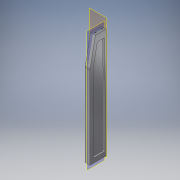
# Autodesk Inventor part: ZcolStiffer
Saved by Autodesk Inventor 2019 (Build 230136000, 136)
## iProperties
Created: 2018-10-03
Part Number: ZcolStiffer
Material: Aluminum 6061-AHC
Document SubType Name: Modeling
Designer: LillaHunden
Density: 2.7 g/cm^3
Appearance: Aluminum - Dark
Mass: 421.378 g
Surface Area: 509.759 cm^2
Volume: 156.066 cm^3
Author: LillaHunden
Autodesk Inventor part; units mm, degrees
ref_plane "YZ Plane" through (0, 0, 0) normal (1, 0, 0) x (0, 1, 0)
ref_plane "XZ Plane" through (0, 0, 0) normal (0, 1, 0) x (-1, 0, 0)
ref_plane "XY Plane" through (0, 0, 0) normal (0, 0, 1) x (1, 0, 0)
ref_plane "Work Plane1" through (0, 0, 0) normal (0, 0, 1) x (1, 0, 0)
sketch "Sketch1" plane through (0, 0, 0) normal (0, 0, 1) x (1, 0, 0)
  line L0 (33.6143, 326.2667) -> (51.0643, 326.2667) construction
  line L1 (0, -13.7333) -> (51.0143, -13.7333) construction
  line L2 (34.8393, 326.2667) -> (49.8393, 326.2667)
  line L3 (49.8393, 326.2667) -> (49.8393, -13.7333)
  line L4 (49.8393, -13.7333) -> (34.8393, -13.7333)
  line L5 (34.8393, -13.7333) -> (34.8393, 326.2667)
  point P0 (0, 0)
  point P1 (51.0143, -13.7333)
  point P2 (42.3393, 326.2667)
  point P3 (42.3393, 326.2667)
  dimension "d0" = 15
  constraints: 8 end point, 2 midpoint, 2 parallel, 1 coincident, 1 horizontal, 1 perpendicular, 1 point on line, 2 other
  measures "d0" distance of L3.end L4.end
extrude "Extrusion1" add sketch "Sketch1" along normal blind 50
sketch "Sketch2" plane through (49.8393, -13.7333, 0) normal (1, 0, 0) x (0, 0, -1)
  line L0 (0, 340) -> (-50, 340) projected
  line L1 (-33.2282, 340) -> (-50, 256.6625)
  line L2 (-50, 0) -> (-50, 340) projected
  line L3 (0, 340) -> (0, 0) projected
  line L4 (-33.2282, 340) -> (-33.2282, 350) construction
  point P0 (0, 13.7333)
  constraints: 2 end point, 1 point on line
extrude "Extrusion2" cut sketch "Sketch2" against normal through all
chamfer "Chamfer2" distance 2 angle 45 1 edges at (42.3393, 242.9292, 50)
sketch "Sketch3" plane through (34.8393, 326.2667, 0) normal (0, 1, 0) x (1, 0, 0)
  point P0 (7.4895, -25.5)
  point P1 (7.4895, -5.5)
hole "Hole1" at (42.3288, 326.2667, 25.5) at (42.3288, 326.2667, 5.5) direction (0, -1, 0) diameter 3.242 depth 12.5366 tip angle 120 thread size "M4x0.7" class "6H" standard "ISO Metric profile"
sketch "Sketch4" plane through (34.8393, -13.7333, 0) normal (-1, 0, 0) x (0, 0, 1)
  line L0 (49.6054, 258.6232) -> (50, 254.6625) construction
  line L1 (49.6054, 258.6232) -> (33.2282, 340) construction
  line L2 (0, 340) -> (33.2282, 340) construction
  line L3 (0, 0) -> (0, 340) construction
  line L4 (0, 0) -> (50, 0) construction
  line L5 (50, 254.6625) -> (50, 0) construction
  line L6 (40, 14) -> (3.5815, 14)
  line L7 (3.5815, 14) -> (5, 320)
  line L8 (27.0527, 320) -> (39.7039, 257.1374)
  line L9 (39.7039, 257.1374) -> (40, 254.1656)
  line L10 (40, 254.1656) -> (40, 14)
  line L11 (5, 320) -> (27.0527, 320)
  line L12 (5, 0) -> (-10, 0) construction
  line L13 (5, 0) -> (5, 340) construction
  line L14 (-10, 340) -> (5, 340) construction
  line L15 (-10, 0) -> (-10, 340) construction
  point P0 (0, 13.7333)
  dimension "d20" = 10
  dimension "d21" = 20
  dimension "d22" = 14
  constraints: 12 end point, 1 horizontal, 1 point on line, 1 other
  measures "d20" distance between parallel lines of L5 L10
  measures "d21" distance between parallel lines of L2 L11
  measures "d22" distance between parallel lines of L6 L4
extrude "Extrusion3" cut sketch "Sketch4" against normal blind 5
fillet "Fillet1" radius 3 4 edges at (37.3393, 0.2667, 3.5815) (37.3393, 0.2667, 40) (37.3393, 306.2667, 5) (37.3393, 306.2667, 27.0527)
ref_plane "Work Plane2" through (42.3393, -13.7333, 0) normal (-1, 0, 0) x (0, 0, 1)
mirror "Mirror2" about plane through (42.3393, -13.7333, 0) normal (-1, 0, 0) of "Extrusion3", "Fillet1"
sketch "Sketch5" plane through (0, 0, 0) normal (0, 0, -1) x (-1, 0, 0)
  circle A0 centre (-42.3893, 30.2667) radius 1.2295 projected
  circle A1 centre (-42.3893, 80.2667) radius 1.2295 projected
  circle A2 centre (-42.3893, 130.2667) radius 1.2295 projected
  circle A3 centre (-42.3893, 180.2667) radius 1.2295 projected
  circle A4 centre (-42.3893, 230.2667) radius 1.2295 projected
  circle A5 centre (-42.3893, 280.2667) radius 1.2295 projected
  circle A6 centre (-42.3893, 305.2667) radius 1.2295 projected
  circle A7 centre (-42.3893, 255.2667) radius 1.2295 projected
  circle A8 centre (-42.3893, 205.2667) radius 1.2295 projected
  circle A9 centre (-42.3893, 155.2667) radius 1.2295 projected
  circle A10 centre (-42.3893, 105.2667) radius 1.2295 projected
  circle A11 centre (-42.3893, 55.2667) radius 1.2295 projected
  circle A12 centre (-42.3893, 5.2667) radius 1.2295 projected
  line L0 (-48.3893, -13.7333) -> (-48.3893, 326.2667) projected
  line L1 (-36.3893, -13.7333) -> (-48.3893, -13.7333) projected
  line L2 (-36.3893, 326.2667) -> (-36.3893, -13.7333) projected
  line L3 (-48.3893, 326.2667) -> (-36.3893, 326.2667) projected
  point P0 (0, 0)
  constraints: 13 coincident
hole "Hole3" at (42.3893, 305.2667, 0) at (42.3893, 280.2667, 0) at (42.3893, 255.2667, 0) at (42.3893, 230.2667, 0) at (42.3893, 205.2667, 0) at (42.3893, 180.2667, 0) at (42.3893, 155.2667, 0) at (42.3893, 130.2667, 0) at (42.3893, 105.2667, 0) at (42.3893, 80.2667, 0) at (42.3893, 55.2667, 0) at (42.3893, 30.2667, 0) at (42.3893, 5.2667, 0) direction (0, 0, 1) diameter 2.459 depth 8.8 tip angle 118 thread size "M3x0.5" class "6H" standard "ISO Metric profile"
body "Solid1"
